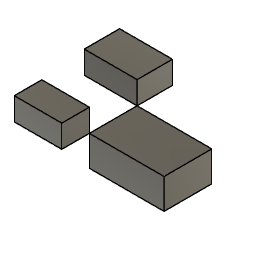
3boxes (Autodesk Fusion 360 design; units mm, degrees)
Autodesk Fusion 360 part; units mm, degrees
sketch "Sketch1" plane through (0, 0, 0) normal (0, 1, 0) x (1, 0, 0)
sketch "Sketch2" plane through (0, 0, 0) normal (0, 0, 1) x (1, 0, 0)
  line L0 (0, 0) -> (49.4434, 0)
  line L1 (49.4434, 0) -> (49.4434, 31.6274)
  line L2 (49.4434, 31.6274) -> (0, 31.6274)
  line L3 (0, 31.6274) -> (0, 0)
  constraint horizontal L0
  constraint vertical L1
  constraint horizontal L2
  constraint vertical L3
  constraint coincident L0.start L3.end
extrude "Extrude1" add sketch "Sketch2" along normal blind 20 makes body 1
sketch "Sketch3" plane through (0, 0, 20) normal (0, 0, 1) x (-1, 0, 0)
  line L0 (0, -31.6274) -> (0, 0)
  line L1 (0, 0) -> (-49.4434, 0)
  line L2 (-49.4434, 0) -> (-49.4434, -31.6274)
  line L3 (-49.4434, -31.6274) -> (0, -31.6274)
  line L4 (0, 0) -> (31.4549, 0)
  line L5 (31.4549, 0) -> (31.4549, 18.2474)
  line L6 (31.4549, 18.2474) -> (0, 18.2474)
  line L7 (0, 18.2474) -> (0, 0)
  line L8 (0, -31.6274) -> (35, -31.6274)
  line L9 (35, -31.6274) -> (35, -55)
  line L10 (35, -55) -> (0, -55)
  line L11 (0, -55) -> (0, -31.6274)
  constraint horizontal L4
  constraint vertical L5
  constraint horizontal L6
  constraint vertical L7
  constraint coincident L0.end L1.start
  constraint horizontal L8
  constraint vertical L9
  constraint horizontal L10
  constraint vertical L11
  constraint coincident L0.start L3.end
extrude "Extrude2" add sketch "Sketch3" along normal blind 15 separate body contours L4 L5 L6 L7 | L8 L9 L10 L11 makes body 2 at (-11.6667, 39.4183, 20) makes body 3 at (-10.485, -12.1649, 20)
